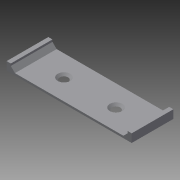
# Autodesk Inventor part: head mount
Saved by Autodesk Inventor 2015 (Build 190159000, 159)
## iProperties
Created: 2019-01-22
Part Number: head mount
Material: Generic
Document SubType Name: Modeling
Designer: Toby
Density: 1 g/cm^3
Appearance: Default
Author: Toby
Autodesk Inventor part; units mm, degrees
ref_plane "YZ Plane" through (0, 0, 0) normal (1, 0, 0) x (0, 1, 0)
ref_plane "XZ Plane" through (0, 0, 0) normal (0, 1, 0) x (-1, 0, 0)
ref_plane "XY Plane" through (0, 0, 0) normal (0, 0, 1) x (1, 0, 0)
sketch "Sketch1" plane through (0, 0, 0) normal (0, 0, 1) x (1, 0, 0)
  line L0 (-30.5603, 10.2886) -> (29.4397, 10.2886)
  line L1 (29.4397, 10.2886) -> (29.4397, -9.7114)
  line L2 (29.4397, -9.7114) -> (-30.5603, -9.7114)
  line L3 (-30.5603, -9.7114) -> (-30.5603, 10.2886)
  point P0 (0, 0)
  dimension "d0" = 60
  dimension "d1" = 20
  constraints: 8 end point, 2 parallel, 1 horizontal, 1 perpendicular
  measures "d0" distance of L0.start L0.end
  measures "d1" distance of L2.end L0.start
extrude "Extrusion1" add sketch "Sketch1" along normal blind 1
sketch "Sketch2" plane through (0, 0, 1) normal (0, 0, 1) x (1, 0, 0)
  line L0 (-30.5603, 10.2886) -> (-30.5603, -9.7114) projected
  line L1 (-30.5603, 10.2886) -> (29.4397, 10.2886) projected
  line L2 (29.4397, -9.7114) -> (29.4397, 10.2886) projected
  point P0 (0, 0)
  point P1 (-13.0603, 0.2886)
  point P2 (11.9397, 0.2886)
  dimension "d4" = 25
  dimension "d5" = 17.5
  dimension "d6" = 10
  dimension "d7" = 10
  dimension "d8" = 17.5
  measures "d4" distance of point (11.94, 0.289) point (-13.06, 0.289)
  measures "d5" distance from line of L0 point (-13.06, 0.289)
  measures "d6" distance from line of L1 point (-13.06, 0.289)
  measures "d7" distance from line of L1 point (11.94, 0.289)
  measures "d8" distance from line of L2 point (11.94, 0.289)
hole "Hole1" at (-13.0603, 0.2886, 1) at (11.9397, 0.2886, 1) direction (0, 0, -1) diameter 3 depth 8 tip angle 118 countersink diameter 6 countersink angle 90
sketch "Sketch3" plane through (0, 0, 1) normal (0, 0, 1) x (1, 0, 0)
  line L0 (-30.5603, 10.2886) -> (-28.5603, 10.2886)
  line L1 (-28.5603, 10.2886) -> (-28.5603, -9.7114)
  line L2 (-28.5603, -9.7114) -> (-30.5603, -9.7114)
  line L3 (-30.5603, -9.7114) -> (-30.5603, 10.2886)
  line L4 (29.4397, 10.2886) -> (27.4397, 10.2886)
  line L5 (27.4397, 10.2886) -> (27.4397, -9.7114)
  line L6 (27.4397, -9.7114) -> (29.4397, -9.7114)
  line L7 (29.4397, -9.7114) -> (29.4397, 10.2886)
  line L8 (-30.5603, -9.7114) -> (29.4397, -9.7114) projected
  point P0 (0, 0)
  dimension "d16" = 2
  dimension "d17" = 2
  constraints: 16 end point, 4 parallel, 2 horizontal, 2 perpendicular, 1 collinear, 1 point on line
  measures "d16" distance between parallel lines of L3 L1
  measures "d17" distance between parallel lines of L7 L5
extrude "Extrusion2" add sketch "Sketch3" along normal blind 3
chamfer "Chamfer1" distance 2 angle 45 2 edges at (-28.5603, 0.2886, 1) (27.4397, 0.2886, 1)
body "Solid1"
